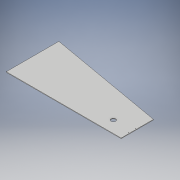
# Autodesk Inventor part: pinball-case-left-wall-outer
Saved by Autodesk Inventor 2017 (Build 210142000, 142)
## iProperties
Created: 2017-02-27
Part Number: pinball-case-left-wall-outer
Material: Generic
Document SubType Name: Modeling
Designer: John
Density: 1 g/cm^3
Appearance: Default
Author: John
Autodesk Inventor part; units mm, degrees
ref_plane "YZ Plane" through (0, 0, 0) normal (1, 0, 0) x (0, 1, 0)
ref_plane "XZ Plane" through (0, 0, 0) normal (0, 1, 0) x (-1, 0, 0)
ref_plane "XY Plane" through (0, 0, 0) normal (0, 0, 1) x (1, 0, 0)
sketch "Sketch1" plane through (0, 0, 0) normal (0, 1, 0) x (-1, 0, 0)
  line L0 (0, 0) -> (-590, 0)
  line L1 (-590, 0) -> (-590, -165.9671)
  line L2 (-590, -165.9671) -> (0, -165.9671)
  line L3 (0, -165.9671) -> (0, 0)
  line L4 (0, -165.9671) -> (0, -270)
  line L5 (0, -270) -> (-590, -165.9671)
  dimension "d0" = 590
  dimension "d28" = 270
  dimension "d29" = 10
  constraints: 12 end point, 2 parallel, 1 horizontal, 1 perpendicular, 1 vertical
  measures "d0" distance of L2.end L1.end
  measures "d28" distance of L0.start L4.end
  measures "d29" angle of L2 L5
extrude "Extrusion1" add sketch "Sketch1" along normal blind 3
sketch "Sketch3" plane through (0, 3, 0) normal (0, 1, 0) x (1, 0, 0)
  circle A0 centre (585.75, 41.75) radius 1.25
  circle A1 centre (585.75, 78.75) radius 1.25
  line L0 (590, 0) -> (590, 165.9671) projected
  line L1 (0, 0) -> (590, 0) projected
  dimension "d15" = 2.5
  dimension "d16" = 4.25
  dimension "d17" = 4.25
  dimension "d18" = 2.5
  dimension "d19" = 41.75
  dimension "d20" = 37
  constraints: 2 centre point
  measures "d15" diameter of A0
  measures "d16" distance from line of L0 A1.centre
  measures "d17" distance from line of L0 A0.centre
  measures "d18" diameter of A1
  measures "d19" distance from line of L1 A0.centre
  measures "d20" distance of A1.centre A0.centre
extrude "Extrusion3" cut sketch "Sketch3" along normal through all both and the other way through all
sketch "Sketch4" plane through (0, 3, 0) normal (0, 1, 0) x (1, 0, 0)
  circle A0 centre (490, 60) radius 12
  line L0 (0, 0) -> (590, 0) projected
  line L1 (590, 0) -> (590, 165.9671) projected
  dimension "d23" = 24
  dimension "d24" = 60
  dimension "d25" = 100
  constraints: 1 centre point
  measures "d23" diameter of A0
  measures "d24" distance from line of L0 A0.centre
  measures "d25" distance from line of L1 A0.centre
extrude "Extrusion4" cut sketch "Sketch4" against normal through all
equation "\"d16\" = d17"
equation "\"d18\" = d15"
body "Solid1"
